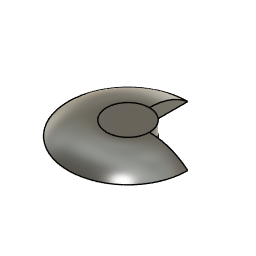
Tapa (Autodesk Fusion 360 design; units mm, degrees)
Autodesk Fusion 360 part; units mm, degrees
sketch "Sketch1" plane through (0, 0, 0) normal (0, 0, 1) x (1, 0, 0)
  circle A0 centre (0, 0) radius 60
  dimension "d1" = 120
  constraint coincident A0.centre origin
  measures "d1" diameter of A0
extrude "Extrude1" add sketch "Sketch1" along normal blind 14
sketch "Sketch2" plane through (0, 0, 0) normal (0, 0, -1) x (1, 0, 0)
  circle A0 centre (0, 0) radius 60
  circle A1 centre (0, 0) radius 5
  dimension "d4" = 10
  constraint coincident A0.centre A1.centre
  measures "d4" diameter of A1
extrude "Extrude2" cut sketch "Sketch2" against normal blind 6 contours A1
sketch "Sketch3" plane through (0, 0, 6) normal (0, 0, -1) x (1, 0, 0)
  circle A0 centre (0, 0) radius 5
  line L0 (4.3301, 2.5) -> (-4.3301, 2.5)
  line L1 (-4.3301, 2.5) -> (-4.3301, -2.5)
  line L2 (-4.3301, -2.5) -> (4.3301, -2.5)
  line L3 (4.3301, -2.5) -> (4.3301, 2.5)
  line L4 (4.3301, 2.5) -> (-4.3301, -2.5) construction
  line L5 (-4.3301, 2.5) -> (4.3301, -2.5) construction
  dimension "d7" = 5
  constraint horizontal L0
  constraint perpendicular L0 L1
  constraint parallel L0 L2
  constraint parallel L1 L3
  constraint coincident L4 A0.centre
  constraint coincident L5 A0.centre
  constraint coincident A0 L0.start
  constraint coincident A0.centre origin
  measures "d7" distance of L0.end L1.end
extrude "Extrude3" cut sketch "Sketch3" against normal blind 5 contours L0 L1 L2 L3
fillet "Fillet1" radius 60 1 edges at (-55.9396, -21.6969, 14)
sketch "Sketch4" plane through (0, 0, 14) normal (0, 0, 1) x (-1, 0, 0)
  circle A0 centre (0, 0) radius 21.4773
  circle A1 centre (0, 0) radius 17.5
  line L0 (0, 0) -> (-60, 0)
  line L1 (0, 0) -> (0, -60)
  line L2 (0, -60) -> (-60, -60)
  line L3 (-60, -60) -> (-60, 0)
  dimension "d12" = 35
  constraint coincident A0.centre A1.centre
  constraint horizontal L0
  constraint perpendicular L0 L1
  constraint perpendicular L1 L2
  constraint perpendicular L0 L3
  measures "d12" diameter of A1
extrude "Extrude4" cut sketch "Sketch4" against normal blind 25 contours A0 L0 L1 L2 L3
